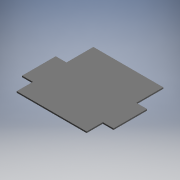
# Autodesk Inventor part: Gen 2.0 rev mecanums base plate
Saved by Autodesk Inventor 2019 (Build 230136000, 136)
## iProperties
Part Number: Gen 2.0 rev mecanums base plate
Material: Generic
Document SubType Name: Modeling
Designer: Delta
Appearance: Default
Author: Delta
Autodesk Inventor part; units mm, degrees
ref_plane "YZ Plane" through (0, 0, 0) normal (1, 0, 0) x (0, 1, 0)
ref_plane "XZ Plane" through (0, 0, 0) normal (0, 1, 0) x (-1, 0, 0)
ref_plane "XY Plane" through (0, 0, 0) normal (0, 0, 1) x (1, 0, 0)
sketch "Sketch1" plane through (0, 0, 0) normal (0, 1, 0) x (-1, 0, 0)
  line L0 (0, 0) -> (431.8, 0)
  line L1 (431.8, 0) -> (431.8, 361.95)
  line L2 (431.8, 361.95) -> (0, 361.95)
  line L3 (0, 361.95) -> (0, 0)
  dimension "d0" = 431.8
  dimension "d1" = 361.95
  constraints: 8 end point, 2 parallel, 1 horizontal, 1 perpendicular
  measures "d0" distance of L1.end L2.end
  measures "d1" distance of L0.end L1.end
extrude "Extrusion1" add sketch "Sketch1" along normal blind 6.35
sketch "Sketch2" plane through (0, 6.35, 0) normal (0, 1, 0) x (1, 0, 0)
  line L0 (-431.8, 0) -> (-431.8, -361.95) projected
  line L1 (-431.8, 0) -> (-381, 0)
  line L2 (-381, 0) -> (-381, -127)
  line L3 (-381, -127) -> (-431.8, -127)
  line L4 (-431.8, -127) -> (-431.8, 0)
  line L5 (-431.8, -361.95) -> (-381, -361.95)
  line L6 (-381, -361.95) -> (-381, -285.75)
  line L7 (-381, -285.75) -> (-431.8, -285.75)
  line L8 (-431.8, -285.75) -> (-431.8, -361.95)
  line L9 (-431.8, -361.95) -> (0, -361.95) projected
  line L10 (0, -361.95) -> (-50.8, -361.95)
  line L11 (-50.8, -361.95) -> (-50.8, -285.75)
  line L12 (-50.8, -285.75) -> (0, -285.75)
  line L13 (0, -285.75) -> (0, -361.95)
  line L14 (0, 0) -> (-50.8, 0)
  line L15 (-50.8, 0) -> (-50.8, -127)
  line L16 (-50.8, -127) -> (0, -127)
  line L17 (0, -127) -> (0, 0)
  dimension "d4" = 127
  dimension "d5" = 50.8
  dimension "d6" = 50.8
  dimension "d7" = 76.2
  constraints: 32 end point, 8 parallel, 4 horizontal, 4 perpendicular, 4 point on line
  measures "d4" distance between parallel lines of L3 L1
  measures "d5" distance between parallel lines of L4 L2
  measures "d6" distance between parallel lines of L17 L15
  measures "d7" distance between parallel lines of L9 L7
extrude "Extrusion2" cut sketch "Sketch2" against normal blind 6.35
body "Solid1"
